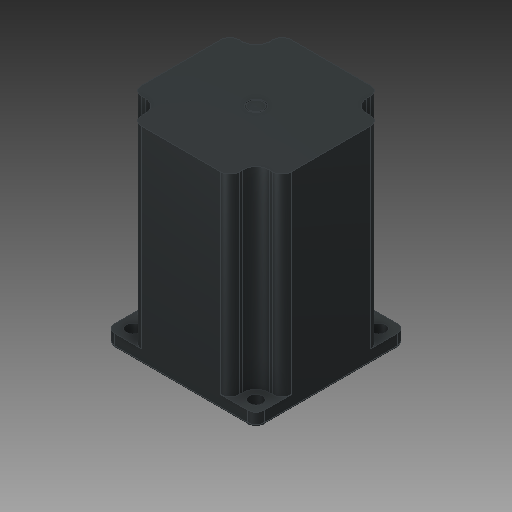
# Autodesk Inventor part: NEMA23
Saved by Autodesk Inventor 2019 (Build 230136000, 136)
## iProperties
Created: 2021-04-25
Part Number: NEMA23
Material: Eisen, Grau
Document SubType Name: Modeling
Designer: Michael Sumper
Density: 7.15 g/cm^3
Appearance: Eisen - Grau
Mass: 1642.7 g
Surface Area: 269.178 cm^2
Volume: 229.748 cm^3
Author: Michael Sumper
Autodesk Inventor part; units mm, degrees
ref_plane "YZ Plane" through (0, 0, 0) normal (1, 0, 0) x (0, 1, 0)
ref_plane "XZ Plane" through (0, 0, 0) normal (0, 1, 0) x (-1, 0, 0)
ref_plane "XY Plane" through (0, 0, 0) normal (0, 0, 1) x (1, 0, 0)
sketch "Skizze1" plane through (0, 0, 0) normal (0, 1, 0) x (-1, 0, 0)
  circle A0 centre (0, 0) radius 19.05
  circle A1 centre (0, 0) radius 5
  dimension "d0" = 38.1
  dimension "d1" = 10
  constraints: 2 centre point, 2 coincident
  measures "d0" diameter of A0
  measures "d1" diameter of A1
extrude "Extrusion1" add sketch "Skizze1" along normal blind 1.524
sketch "Skizze2" plane through (0, 1.524, 0) normal (0, 1, 0) x (1, 0, 0)
  line L0 (28.575, -28.575) -> (-28.575, -28.575)
  line L1 (-28.575, -28.575) -> (-28.575, 28.575)
  line L2 (-28.575, 28.575) -> (28.575, 28.575)
  line L3 (28.575, 28.575) -> (28.575, -28.575)
  line L4 (28.575, -28.575) -> (-28.575, 28.575) construction
  line L5 (-28.575, -28.575) -> (28.575, 28.575) construction
  line L6 (23.5, -23.5) -> (-23.5, -23.5) construction
  line L7 (-23.5, -23.5) -> (-23.5, 23.5) construction
  line L8 (-23.5, 23.5) -> (23.5, 23.5) construction
  line L9 (23.5, 23.5) -> (23.5, -23.5) construction
  line L10 (23.5, -23.5) -> (-23.5, 23.5) construction
  line L11 (-23.5, -23.5) -> (23.5, 23.5) construction
  circle A0 centre (-23.5, -23.5) radius 2.54
  circle A1 centre (-23.5, 23.5) radius 2.54
  circle A2 centre (23.5, 23.5) radius 2.54
  circle A3 centre (23.5, -23.5) radius 2.54
  circle A4 centre (0, 0) radius 3.175
  dimension "d4" = 57.15
  dimension "d5" = 57.15
  dimension "d6" = 47
  dimension "d7" = 47
  dimension "d8" = 5.08
  dimension "d9" = 5.08
  dimension "d10" = 5.08
  dimension "d11" = 5.08
  dimension "d43" = 6.35
  constraints: 24 end point, 5 centre point, 5 coincident, 4 midpoint, 4 parallel, 2 horizontal, 2 perpendicular
  measures "d4" distance of L1.end L2.end
  measures "d5" distance of L0.end L1.end
  measures "d6" distance of L7.end L8.end
  measures "d7" distance of L6.end L7.end
  measures "d8" diameter of A0
  measures "d9" diameter of A1
  measures "d10" diameter of A2
  measures "d11" diameter of A3
  measures "d43" diameter of A4
extrude "Extrusion2" add sketch "Skizze2" along normal blind 5.08 contours L0 L1 L2 L3 | A4
sketch "Skizze3" plane through (0, 6.604, 0) normal (0, 1, 0) x (1, 0, 0)
  line L0 (-28.575, -28.575) -> (-28.575, 28.575) projected
  line L1 (-28.575, -28.575) -> (-18.644, -28.575) construction
  line L2 (-18.644, -28.575) -> (-18.644, -23.622)
  line L3 (-23.622, -18.644) -> (-28.575, -18.644)
  line L4 (-28.575, -18.644) -> (-28.575, -28.575) construction
  line L5 (-28.575, 28.575) -> (-18.644, 28.575) construction
  line L6 (-18.644, 28.575) -> (-18.644, 23.622)
  line L7 (-23.622, 18.644) -> (-28.575, 18.644)
  line L8 (-28.575, 18.644) -> (-28.575, 28.575) construction
  line L9 (28.575, 28.575) -> (28.575, -28.575) construction
  line L10 (28.575, 28.575) -> (18.644, 28.575) construction
  line L11 (18.644, 28.575) -> (18.644, 23.622)
  line L12 (23.622, 18.644) -> (28.575, 18.644)
  line L13 (28.575, 18.644) -> (28.575, 28.575) construction
  line L14 (28.575, -28.575) -> (18.644, -28.575) construction
  line L15 (18.644, -28.575) -> (18.644, -23.622)
  line L16 (23.622, -18.644) -> (28.575, -18.644)
  line L17 (28.575, -18.644) -> (28.575, -28.575) construction
  arc A0 (-18.644, -23.622) -> (-23.622, -18.644) centre (-23.622, -23.622) ccw
  line L18 (-28.575, 28.575) -> (-28.575, -28.575) projected
  line L19 (-28.575, -28.575) -> (28.575, -28.575) projected
  line L20 (28.575, 28.575) -> (-28.575, 28.575) projected
  arc A1 (-23.622, 18.644) -> (-18.644, 23.622) centre (-23.622, 23.622) ccw
  arc A2 (23.622, -18.644) -> (18.644, -23.622) centre (23.622, -23.622) ccw
  arc A3 (18.644, 23.622) -> (23.622, 18.644) centre (23.622, 23.622) ccw
  line L21 (-18.644, -28.575) -> (18.644, -28.575)
  line L22 (28.575, -28.575) -> (-28.575, -28.575) projected
  line L23 (28.575, -18.644) -> (28.575, 18.644)
  line L24 (18.644, 28.575) -> (-18.644, 28.575)
  line L25 (-28.575, 28.575) -> (28.575, 28.575) projected
  line L26 (-28.575, 18.644) -> (-28.575, -18.644)
  point P0 (0, 0)
  point P1 (-18.644, -18.644)
  point P2 (-18.644, 18.644)
  point P3 (18.644, 18.644)
  point P4 (18.644, -18.644)
  dimension "d14" = 9.931
  dimension "d15" = 9.931
  dimension "d16" = 9.931
  dimension "d17" = 9.931
  dimension "d18" = 9.931
  dimension "d19" = 9.931
  dimension "d20" = 9.931
  dimension "d21" = 9.931
  dimension "d22" = 4.978
  dimension "d23" = 4.978
  dimension "d24" = 4.978
  dimension "d25" = 4.978
  constraints: 40 end point, 8 parallel, 8 point on circle, 8 point on line, 8 tangent, 5 perpendicular, 4 centre point, 4 horizontal, 3 collinear
  measures "d14" distance of L3.end point (-18.644, -18.644)
  measures "d15" distance of point (-18.644, -18.644) L1.end
  measures "d16" distance of point (-18.644, 18.644) L7.end
  measures "d17" distance of L5.end point (-18.644, 18.644)
  measures "d18" distance of L12.end point (18.644, 18.644)
  measures "d19" distance of point (18.644, 18.644) L10.end
  measures "d20" distance of point (18.644, -18.644) L16.end
  measures "d21" distance of L14.end point (18.644, -18.644)
  measures "d22" radius of A0
  measures "d23" radius of A1
  measures "d24" radius of A2
  measures "d25" radius of A3
extrude "Extrusion3" add sketch "Skizze3" along normal blind 73.66 contours L0 L7 A1 L6 L20 L11 A3 L12 L23 L16 A2 L15 L19 L2 A0 L3
fillet "Rundung1" radius 3.556 8 edges at (18.644, 43.434, 28.575) (28.575, 43.434, 18.644) (28.575, 43.434, -18.644) (18.644, 43.434, -28.575) (-18.644, 43.434, -28.575) (-28.575, 43.434, -18.644) (-28.575, 43.434, 18.644) (-18.644, 43.434, 28.575)
sketch "Skizze4" plane through (0, 0, 0) normal (0, -1, 0) x (1, 0, 0)
  circle A0 centre (0, 0) radius 19.05 projected
  circle A1 centre (0, 0) radius 20.32
  dimension "d29" = 1.27
  constraints: 1 centre point
  measures "d29" radial gap between concentric circles of A0 A1
extrude "Extrusion4" cut sketch "Skizze4" against normal blind 2.032
fillet "Rundung2" radius 3.175 4 edges at (28.575, 4.064, -28.575) (-28.575, 4.064, -28.575) (-28.575, 4.064, 28.575) (28.575, 4.064, 28.575)
sketch "Skizze5" plane through (0, 80.264, 0) normal (0, 1, 0) x (1, 0, 0)
  circle A0 centre (0, 0) radius 3.175
  dimension "d33" = 6.35
  constraints: 1 centre point, 1 coincident
  measures "d33" diameter of A0
extrude "Extrusion5" add sketch "Skizze5" against normal blind 99.314 separate body
sketch "Skizze6" plane through (0, -19.05, 0) normal (0, -1, 0) x (1, 0, 0)
  circle A0 centre (0, 0) radius 3.175 projected
  line L0 (2.4512, -2.018) -> (2.8362, 1.427)
  circle A1 centre (0, 0) radius 3.175 projected
  dimension "d36" = 3.445
  constraints: 2 end point, 1 point on circle, 3 other
  measures "d36" vertical distance of L0.start L0.end
extrude "Extrusion6" cut sketch "Skizze6" against normal blind 15 contours A0 L0 picked at (2.7112, -0.6661) bodies 2
chamfer "Fase1" distance 0.5 angle 45 3 edges at (-3.1554, -19.05, 0.3526) (2.6437, -19.05, -0.2955) (-3.175, 80.264, 0)
fillet "Rundung3" radius 0.991 8 edges at (27.6451, 1.524, -27.6451) (28.575, 1.524, 0) (27.6451, 1.524, 27.6451) (0, 1.524, 28.575) (-27.6451, 1.524, 27.6451) (-28.575, 1.524, 0) (-27.6451, 1.524, -27.6451) (0, 1.524, -28.575)
extrude "Extrusion7" cut sketch "Skizze2" along normal blind 100 contours A4 bodies 1
sketch "Skizze7" plane through (0, 1.524, 0) normal (0, -1, 0) x (1, 0, 0)
  circle A0 centre (23.5, 23.5) radius 2.54 projected
  circle A1 centre (23.5, -23.5) radius 2.54 projected
  circle A2 centre (-23.5, -23.5) radius 2.54 projected
  circle A3 centre (-23.5, 23.5) radius 2.54 projected
  point P0 (0, 0)
extrude "Extrusion8" add sketch "Skizze7" against normal blind 5.08 bodies 1
hole "Bohrung1" at (23.5, 1.524, -23.5) at (23.5, 1.524, 23.5) at (-23.5, 1.524, 23.5) at (-23.5, 1.524, -23.5) direction (0, -1, 0) diameter 5.08 end through all start extended yes bodies 1
